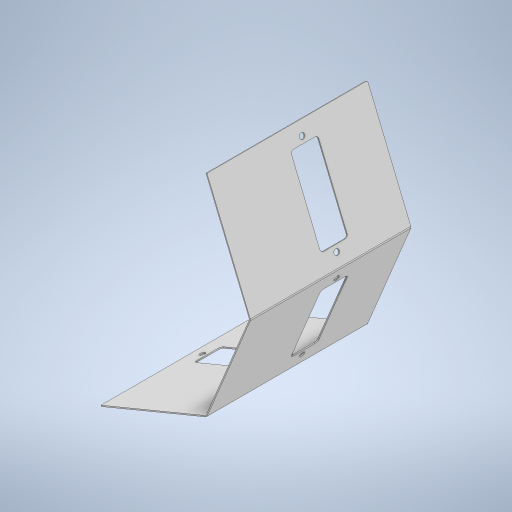
# Autodesk Inventor part: ДМС 100 Барабан Лист №3 ПВГ
Saved by Autodesk Inventor 2024.2 (Build 282272000, 272)
## iProperties
Created: 2024-04-28
Part Number: ДМС 100 Барабан Лист №3 ПВГ
Material: Generic
Document SubType Name: Sheet Metal
Designer: pokla
Density: 1 g/cm^3
Appearance: Default
Sheet Metal Rule: Default
Flat Pattern Width: 29.375 cm
Flat Pattern Length: 62.4873 cm
Flat Pattern Area: 1835.56 cm^2
Sheet Metal Width: 293,750 mm
Sheet Metal Length: 624,873 mm
Sheet Metal Area: 183556,345 mm^2
Author: pokla
Autodesk Inventor part; units mm, degrees
ref_plane "YZ Plane" through (0, 0, 0) normal (1, 0, 0) x (0, 1, 0)
ref_plane "XZ Plane" through (0, 0, 0) normal (0, 1, 0) x (-1, 0, 0)
ref_plane "XY Plane" through (0, 0, 0) normal (0, 0, 1) x (1, 0, 0)
sketch "Sketch2" plane through (0, 0, 0) normal (0, 0, 1) x (1, 0, 0)
  line L0 (0, 273.845227) -> (193.637817, 193.637817) construction
  line L1 (193.637817, 193.637817) -> (273.845227, 0) construction
  line L2 (273.845227, 0) -> (193.637817, -193.637817) construction
  line L3 (193.637817, -193.637817) -> (0, -273.845227) construction
  line L4 (0, -273.845227) -> (-193.637817, -193.637817) construction
  line L5 (-193.637817, -193.637817) -> (-273.845227, 0) construction
  line L6 (-273.845227, 0) -> (-193.637817, 193.637817) construction
  line L7 (-193.637817, 193.637817) -> (0, 273.845227) construction
  line L8 (193.982232, 192.806325) -> (273.211176, 1.530734)
  line L9 (273.211176, -1.530734) -> (194.271867, -192.107083)
  arc A0 (273.211176, -1.530734) -> (273.211176, 1.530734) centre (269.515658, 0) ccw
  line L10 (192.107083, -194.271867) -> (0.831492, -273.500812)
  arc A1 (192.107083, -194.271867) -> (194.271867, -192.107083) centre (190.576349, -190.576349) ccw
  point P0 (0, 0)
  point P1 (0, 0)
  dimension "d56" = 506
  dimension "d58" = 4
  dimension "d69" = 0.9
  dimension "d70" = 4
  dimension "d71" = 0.9
  measures "d56" distance between parallel lines of L6 L2
  measures "d58" radius of A0
  measures "d69" distance of L3.end L10.end
  measures "d70" radius of A1
  measures "d71" distance of L0.end L8.start
contour flange "Contour Flange2" sketch "Sketch2" thickness 2 bend radius 2 width 2006 along (0, 0, -1) mid plane no both sides no wall seen from (233.596704, 97.168529, 0) lies toward (-0.9238795, -0.3826834, 0) curves L8 A0 L9 A1 L10
bend "Bend2"
corner "Corner2"
sketch "Sketch10" plane through (194.271867, -192.107083, 0) normal (0.9238795, -0.3826834, 0) x (0, 0, -1)
  line L0 (1103, 175.639177) -> (1153, 175.639177)
  line L1 (1153, 175.639177) -> (1153, 30.639177)
  line L2 (1153, 30.639177) -> (1103, 30.639177)
  line L3 (1103, 30.639177) -> (1103, 175.639177)
  circle A0 centre (1128, 185.639177) radius 5
  circle A1 centre (1128, 20.639177) radius 5
  line L4 (1103, 103.139177) -> (1153, 103.139177) construction
  line L5 (2006, 206.278354) -> (2006, 0) construction
  line L6 (2006, 206.278354) -> (0, 206.278354) construction
  point P0 (0, 103.139177)
  point P1 (1128, 175.639177)
  point P2 (2006, 103.139177)
  point P3 (1003, 206.278354)
  point P4 (1003, 206.278354)
  dimension "d107" = 145
  dimension "d108" = 50
  dimension "d109" = 10
  dimension "d110" = 10
  dimension "d118" = 125
  constraints: 10 end point, 6 midpoint, 2 centre point, 2 parallel, 1 horizontal, 1 horizontal alignment, 1 perpendicular, 1 vertical alignment, 1 other
  measures "d107" distance of L0.end L1.end
  measures "d108" distance of L0.start L0.end
  measures "d109" diameter of A0
  measures "d110" distance from line of L0 A0.centre
  measures "d118" horizontal distance of point (1003, 206.278) point (1128, 175.639)
extrude "Extrusion4" cut sketch "Sketch10" against normal up to surface (2 mm away)
fillet "Fillet1" radius 5 4 edges at (260.5622, -29.455, -1153) (260.5622, -29.455, -1103) (205.0731, -163.4175, -1103) (205.0731, -163.4175, -1153)
pattern_circular "Circular Pattern1" count 3 over 90 about axis through (0, 0, -10) along (0, 0, 1) of "Extrusion4", "Fillet1" both ways yes
pattern_linear "Rectangular Pattern2" count 8 spacing 250 along (0, 0, 1) of "Extrusion4", "Fillet1", "Circular Pattern1" first direction both ways yes
chamfer "Corner Chamfer1" distance 2 angle 45 1 edges at (193.0584, 192.4236, -2006)
sketch "Sketch11" plane through (0, 0, 0) normal (0, 1, 0) x (-1, 0, 0)
  line L0 (300, 0) -> (-300, 0)
  line L1 (-300, 0) -> (-300, -1712.25)
  line L2 (-300, -1712.25) -> (300, -1712.25)
  line L3 (300, -1712.25) -> (300, 0)
  point P0 (0, 0)
  point P1 (0, 0)
  dimension "d125" = 600
  dimension "d126" = 1712.25
  constraints: 8 end point, 2 parallel, 1 coincident, 1 horizontal, 1 midpoint, 1 perpendicular
  measures "d125" distance of L2.end L1.end
  measures "d126" distance of L1.end L0.end
extrude "Extrusion5" cut sketch "Sketch11" along normal mid plane 600
equation "\"d118\" = Отступ_окна_от_середины"
equation "\"d56\" = Барабан_габарит_по_кассетам"
equation "\"d58\" = BendRadius + Thickness"
equation "\"d69\" = Барабан_отступ_развертки"
equation "\"d70\" = BendRadius + Thickness"
equation "\"d71\" = Барабан_отступ_развертки"
equation "\"d107\" = Длина_окна_барабан"
equation "\"d108\" = Ширина_окна_барабан"
equation "\"d109\" = Диам_шпильки_под_кассету"
equation "\"d25\" = Thickness"
equation "\"d26\" = BendReliefWidth"
equation "\"d27\" = BendReliefDepth"
equation "\"d28\" = MinimumRemnant"
equation "\"d29\" = TransitionRadius"
equation "\"d30\" = Барабан_длина_листа"
equation "\"d31\" = BendRadius"
equation "\"d33\" = CornerReliefSize"
equation "\"d34\" = GapSize"
equation "\"d35\" = JacobiRadiusSize"
equation "\"BendRadius\" = Thickness"
equation "\"BendReliefWidth\" = Thickness"
equation "\"BendReliefDepth\" = 0.5 * Thickness"
equation "\"CornerReliefSize\" = 4 * Thickness"
equation "\"MinimumRemnant\" = 2 * Thickness"
equation "\"TransitionRadius\" = BendRadius"
equation "\"JacobiRadiusSize\" = BendRadius"
equation "\"GapSize\" = Thickness"
equation "\"Барабан_габарит_по_кассетам\" = 506"
equation "\"Thickness\" = 2"
equation "\"Барабан_отступ_развертки\" = 0.9"
equation "\"Длина_окна_барабан\" = 145"
equation "\"Ширина_окна_барабан\" = 50"
equation "\"Диам_шпильки_под_кассету\" = 10"
equation "\"Барабан_длина_листа\" = 2006"
equation "\"Отступ_окна_от_середины\" = 125"
body "Solid2"
